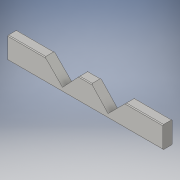
# Autodesk Inventor part: Lower Decoration
Saved by Autodesk Inventor 2016 (Build 200138000, 138)
## iProperties
Created: 2016-07-05
Part Number: Lower Decoration
Material: Generic
Document SubType Name: Modeling
Designer: kurti
Density: 1 g/cm^3
Appearance: Default
Author: kurti
Autodesk Inventor part; units mm, degrees
ref_plane "YZ Plane" through (0, 0, 0) normal (1, 0, 0) x (0, 1, 0)
ref_plane "XZ Plane" through (0, 0, 0) normal (0, 1, 0) x (-1, 0, 0)
ref_plane "XY Plane" through (0, 0, 0) normal (0, 0, 1) x (1, 0, 0)
sketch "Sketch1" plane through (0, 0, 0) normal (0, 0, 1) x (1, 0, 0)
  line L0 (0, 0) -> (635, 0)
  line L1 (635, 0) -> (635, 88.9)
  line L2 (0, 0) -> (0, 88.9)
  line L3 (0, 88.9) -> (152.4, 88.9)
  line L4 (635, 88.9) -> (482.6, 88.9)
  line L5 (482.6, 88.9) -> (152.4, 88.9) construction
  line L6 (317.5, 88.9) -> (292.1, 88.9)
  line L7 (317.5, 88.9) -> (342.9, 88.9)
  line L8 (482.6, 88.9) -> (410.758, 17.058)
  line L9 (482.6, 88.9) -> (584.2, 88.9) construction
  line L10 (342.9, 88.9) -> (410.758, 17.058)
  line L11 (152.4, 88.9) -> (224.242, 17.058)
  line L12 (152.4, 88.9) -> (254, 88.9) construction
  line L13 (224.242, 17.058) -> (292.1, 88.9)
  dimension "d0" = 635
  dimension "d1" = 88.9
  dimension "d2" = 88.9
  dimension "d3" = 152.4
  dimension "d4" = 152.4
  dimension "d5" = 25.4
  dimension "d6" = 25.4
  dimension "d7" = 101.6
  dimension "d8" = 135
  dimension "d9" = 101.6
  dimension "d10" = 45
  constraints: 28 end point, 4 horizontal, 2 equal length, 2 perpendicular, 2 point on line, 1 midpoint, 1 vertical
  measures "d0" distance of L0.start L0.end
  measures "d1" distance of L0.end L1.end
  measures "d2" distance of L0.start L2.end
  measures "d3" distance of L2.end L3.end
  measures "d4" distance of L1.end L4.end
  measures "d5" distance of L6.start L6.end
  measures "d6" distance of L6.start L7.end
  measures "d7" distance of L4.end L8.end
  measures "d8" angle of L8 L9
  measures "d9" distance of L3.end L11.end
  measures "d10" angle of L11 L12
extrude "Extrusion1" add sketch "Sketch1" along normal blind 38.1
fillet "Fillet1" radius 3.175 8 edges at (317.5, 0, 0) (76.2, 88.9, 0) (304.8, 88.9, 0) (558.8, 88.9, 0) (558.8, 88.9, 38.1) (304.8, 88.9, 38.1) (76.2, 88.9, 38.1) (317.5, 0, 38.1)
body "Solid1"
